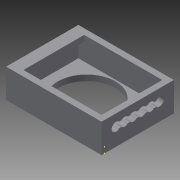
# Autodesk Inventor part: Sensor_Bracket
Saved by Autodesk Inventor 2015 (Build 190159000, 159)
## iProperties
Created: 2017-03-13
Part Number: Sensor_Bracket
Material: Generic
Document SubType Name: Modeling
Designer: ks2101
Density: 1 g/cm^3
Appearance: Default
Author: ks2101
Autodesk Inventor part; units mm, degrees
ref_plane "YZ Plane" through (0, 0, 0) normal (1, 0, 0) x (0, 1, 0)
ref_plane "XZ Plane" through (0, 0, 0) normal (0, 1, 0) x (-1, 0, 0)
ref_plane "XY Plane" through (0, 0, 0) normal (0, 0, 1) x (1, 0, 0)
sketch "Sketch1" plane through (0, 0, 0) normal (0, 0, 1) x (1, 0, 0)
  point P0 (0, 0)
sketch "Sketch2" plane through (0, 0, 0) normal (0, 1, 0) x (-1, 0, 0)
  point P0 (0, 0)
sketch "Sketch3" plane through (0, 0, 0) normal (0, 0, 1) x (1, 0, 0)
  point P0 (0, 0)
sketch "Sketch4" plane through (0, 0, 0) normal (0, 1, 0) x (-1, 0, 0)
  line L0 (33, 1) -> (0, 1)
  line L1 (0, 1) -> (0, -24)
  line L2 (0, -24) -> (33, -24)
  line L3 (33, -24) -> (33, 1)
  dimension "d0" = 33
  dimension "d2" = 25
  constraints: 8 end point, 2 parallel, 1 horizontal, 1 perpendicular
  measures "d0" distance of L1.end L2.end
  measures "d2" distance of L0.end L1.end
extrude "Extrusion1" add sketch "Sketch4" along normal blind 2
sketch "Sketch8" plane through (0, 2, 0) normal (0, 1, 0) x (1, 0, 0)
  line L0 (-0.0049, 24) -> (-32.9741, 24) projected
  line L1 (0, 0) -> (-2, 0)
  line L2 (-2, 0) -> (-2, 24)
  line L3 (-2, 24) -> (0, 24)
  line L4 (0, 24) -> (0, 0)
  dimension "d18" = 2
  constraints: 8 end point, 2 parallel, 1 horizontal, 1 perpendicular, 1 point on line
  measures "d18" distance of L2.end L3.end
sketch "Sketch13" plane through (0, 2, 0) normal (0, 1, 0) x (1, 0, 0)
  point P0 (0, 0)
sketch "Sketch14" plane through (0, 2, 0) normal (0, 1, 0) x (1, 0, 0)
  point P0 (0, 0)
extrude "Extrusion9" add sketch "Sketch8" along normal blind 8
sketch "Sketch15" plane through (0, 2, 0) normal (0, 1, 0) x (1, 0, 0)
  line L0 (-33, -1) -> (0, -1)
  line L1 (0, -1) -> (0, 1)
  line L2 (0, 1) -> (-33, 1)
  line L3 (-33, 1) -> (-33, -1)
  point P0 (0, 0)
  dimension "d32" = 2
  constraints: 8 end point, 2 parallel, 1 horizontal, 1 perpendicular
  measures "d32" distance of L2.end L0.start
extrude "Extrusion10" add sketch "Sketch15" along normal blind 8
sketch "Sketch16" plane through (0, 2, 0) normal (0, 1, 0) x (1, 0, 0)
  line L0 (0, 0) -> (0, 24) projected
  line L1 (-33, 24) -> (0, 24)
  line L2 (0, 24) -> (0, 21.9991)
  line L3 (0, 21.9991) -> (-33, 21.9991)
  line L4 (-33, 21.9991) -> (-33, 24)
  constraints: 8 end point, 2 parallel, 1 horizontal, 1 perpendicular, 1 point on line
extrude "Extrusion11" add sketch "Sketch16" along normal blind 8
sketch "Sketch17" plane through (0, 2, 0) normal (0, 1, 0) x (1, 0, 0)
  line L0 (0, 24) -> (-33, 24) projected
  line L1 (-33, -1) -> (-31.0023, -1)
  line L2 (-31.0023, -1) -> (-31.0023, 24)
  line L3 (-31.0023, 24) -> (-33, 24)
  line L4 (-33, 24) -> (-33, -1)
  point P0 (0, 0)
  constraints: 8 end point, 2 parallel, 1 horizontal, 1 perpendicular, 1 point on line
extrude "Extrusion12" add sketch "Sketch17" along normal blind 8
sketch "Sketch18" plane through (-31.0023, 2, -1) normal (1, 0, 0) x (0, 0, -1)
  line L0 (23, -2) -> (23, 8) projected
  line L1 (-2, 8) -> (23, 8)
  line L2 (23, 8) -> (23, 5.9835)
  line L3 (23, 5.9835) -> (-2, 5.9835)
  line L4 (-2, 5.9835) -> (-2, 8)
  point P0 (-1, -2)
  constraints: 8 end point, 2 parallel, 1 horizontal, 1 perpendicular, 1 point on line
extrude "Extrusion13" add sketch "Sketch18" along normal blind 2
sketch "Sketch19" plane through (0, 0, 1) normal (1, 0, 0) x (0, 0, -1)
  point P0 (1, 0)
sketch "Sketch20" plane through (0, 0, 1) normal (1, 0, 0) x (0, 0, -1)
  circle A0 centre (5, 6) radius 1.5
  line L0 (0, 0) -> (25, 0) projected
  line L1 (0, 0) -> (0, 10) projected
  circle A1 centre (8, 6) radius 1.5
  circle A2 centre (11, 6) radius 1.4979
  circle A3 centre (14, 6) radius 1.5
  circle A4 centre (17, 6) radius 1.5
  circle A5 centre (20, 6) radius 1.5
  line L2 (25, 0) -> (25, 10) projected
  point P0 (1, 0)
  dimension "d41" = 6
  dimension "d42" = 5
  dimension "d43" = 3
  dimension "d44" = 3
  dimension "d45" = 3
  dimension "d46" = 3
  dimension "d47" = 3
  dimension "d48" = 3
  dimension "d49" = 3
  dimension "d50" = 3
  dimension "d51" = 3
  dimension "d52" = 3
  dimension "d60" = 5
  constraints: 6 centre point
  measures "d41" distance from line of A0.centre L0
  measures "d42" distance from line of L1 A0.centre
  measures "d43" distance of A1.centre A0.centre
  measures "d44" diameter of A0
  measures "d45" diameter of A1
  measures "d46" distance of A1.centre A2.centre
  measures "d47" diameter of A3
  measures "d48" diameter of A4
  measures "d49" diameter of A5
  measures "d50" distance of A3.centre A2.centre
  measures "d51" distance of A4.centre A3.centre
  measures "d52" distance of A5.centre A4.centre
  measures "d60" distance from line of L2 A5.centre
hole "Hole1" at (0, 6, -4) at (0, 6, -7) at (0, 6, -10) at (0, 6, -13) at (0, 6, -16) at (0, 6, -19) direction (-1, 0, 0) diameter 3 depth 2 tip angle 118
sketch "Sketch21" plane through (-2, 2, -1) normal (-1, 0, 0) x (0, 0, 1)
  point P0 (1, -2)
sketch "Sketch22" plane through (-2, 2, -1) normal (-1, 0, 0) x (0, 0, 1)
  point P0 (1, -2)
sketch "Sketch23" plane through (0, 0, 1) normal (1, 0, 0) x (0, 0, -1)
  line L0 (5, 7) -> (20.6591, 7)
  line L1 (20.6591, 7) -> (20.6591, 5)
  line L2 (20.6591, 5) -> (5, 5)
  line L3 (5, 5) -> (5, 7)
  arc A0 (12.5, 6) -> (9.5, 6) centre (11, 6) ccw projected
  arc A1 (9.5, 6) -> (12.5, 6) centre (11, 6) ccw projected
  point P0 (1, 0)
  dimension "d62" = 0.5
  dimension "d64" = 0.5
  constraints: 8 end point, 2 parallel, 1 horizontal, 1 perpendicular
  measures "d62" distance edge to line of A1 L2
  measures "d64" distance edge to line of A0 L0
extrude "Extrusion14" cut sketch "Sketch23" against normal blind 9.525 contours L0 A0 A1 L2 L3 | L0 A0 A1 L2 | L0 L1 L2 A1 A0
sketch "Sketch24" plane through (0, 0, 0) normal (0, -1, 0) x (1, 0, 0)
  point P0 (0, 0)
sketch "Sketch26" plane through (0, 0, 0) normal (0, -1, 0) x (1, 0, 0)
  point P0 (0, 0)
sketch "Sketch27" plane through (0, 0, 0) normal (0, -1, 0) x (1, 0, 0)
  circle A0 centre (-17.6464, -11.4968) radius 10
  line L0 (-33, 1) -> (0, 1) projected
  line L1 (0, -24) -> (-33, -24) projected
  point P0 (0, 0)
  dimension "d69" = 20
  dimension "d70" = 12.4968
  dimension "d71" = 12.5032
  constraints: 1 centre point
  measures "d69" diameter of A0
  measures "d70" distance from line of A0.centre L0
  measures "d71" distance from line of A0.centre L1
hole "Hole2" at (-17.6464, 0, -11.4968) direction (0, 1, 0) diameter 20 depth 2 tip angle 118
body "Solid1"
